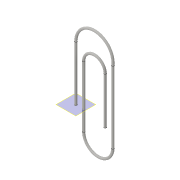
# Autodesk Inventor part: Paperclip
Saved by Autodesk Inventor 2016 (Build 200138000, 138)
## iProperties
Created: 2016-01-26
Part Number: Paperclip
Material: Generic
Document SubType Name: Modeling
Designer: 301278
Density: 1 g/cm^3
Appearance: Default
Author: 301278
Autodesk Inventor part; units mm, degrees
ref_plane "YZ Plane" through (0, 0, 0) normal (1, 0, 0) x (0, 1, 0)
ref_plane "XZ Plane" through (0, 0, 0) normal (0, 1, 0) x (-1, 0, 0)
ref_plane "XY Plane" through (0, 0, 0) normal (0, 0, 1) x (1, 0, 0)
sketch "Sketch1" plane through (0, 0, 0) normal (0, 0, 1) x (1, 0, 0)
  line L0 (20.3826, 0) -> (20.3826, 51.3513)
  arc A0 (20.3826, 51.3513) -> (-3.3847, 51.3513) centre (8.4989, 51.3513) ccw
  line L1 (-3.3847, 51.3513) -> (-3.3847, -15.8811)
  arc A1 (-3.3847, -15.8811) -> (28.8156, -15.8811) centre (12.7154, -15.8811) ccw
  line L2 (28.8156, -15.8811) -> (28.8156, 63.235)
  arc A2 (28.8156, 63.235) -> (-11.9901, 65.8875) centre (8.4989, 65.8875) ccw
  line L3 (-11.9901, 65.8875) -> (-11.9901, 5.4603)
  point P0 (0, 0)
  constraints: 8 end point, 6 point on circle, 4 vertical, 3 centre point
ref_plane "Work Plane1" through (-11.9901, 5.4603, 0) normal (0, -1, 0) x (1, 0, 0)
sketch "Sketch2" plane through (-11.9901, 5.4603, 0) normal (0, -1, 0) x (1, 0, 0)
  circle A0 centre (0, 0) radius 1.27
  point P0 (11.9901, 0)
  dimension "d0" = 2.54
  constraints: 1 centre point
  measures "d0" diameter of A0
sweep "Sweep1" add profiles "Sketch2" path "Sketch1"
body "Solid1"
